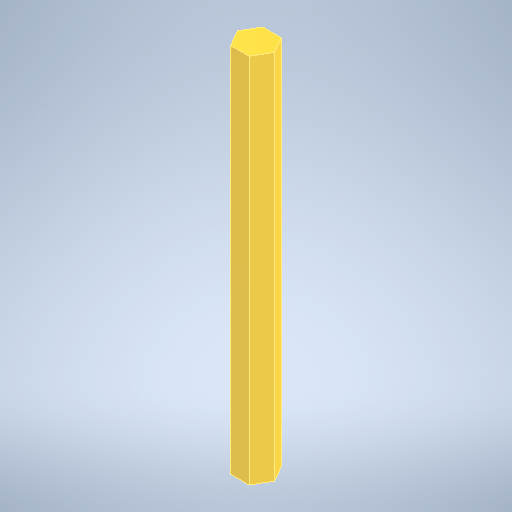
# Autodesk Inventor part: Viga
Saved by Autodesk Inventor 2025.2 (Build 292293000, 293)
## iProperties
Created: 2025-11-06
Part Number: Viga
Material: Genérico
Document SubType Name: Modeling
Designer: Dax
Density: 1 g/cm^3
Appearance: Brillante - Oro
Author: Dax
Autodesk Inventor part; units mm, degrees
ref_plane "YZ Plane" through (0, 0, 0) normal (1, 0, 0) x (0, 1, 0)
ref_plane "XZ Plane" through (0, 0, 0) normal (0, 1, 0) x (-1, 0, 0)
ref_plane "XY Plane" through (0, 0, 0) normal (0, 0, 1) x (1, 0, 0)
sketch "Boceto1" plane through (0, 0, 0) normal (0, 1, 0) x (-1, 0, 0)
  line L0 (2.5, 0) -> (1.25, -2.1651)
  line L1 (1.25, -2.1651) -> (-1.25, -2.1651)
  line L2 (-1.25, -2.1651) -> (-2.5, 0)
  line L3 (-2.5, 0) -> (-1.25, 2.1651)
  line L4 (-1.25, 2.1651) -> (1.25, 2.1651)
  line L5 (1.25, 2.1651) -> (2.5, 0)
  point P0 (0, 0)
  point P1 (0, 0)
  dimension "d0" = 2.5
  constraints: 12 end point, 1 coincident, 13 other
  measures "d0" distance of point (0, 0) L0.start
extrude "Extrusión1" add sketch "Boceto1" along normal blind 50
